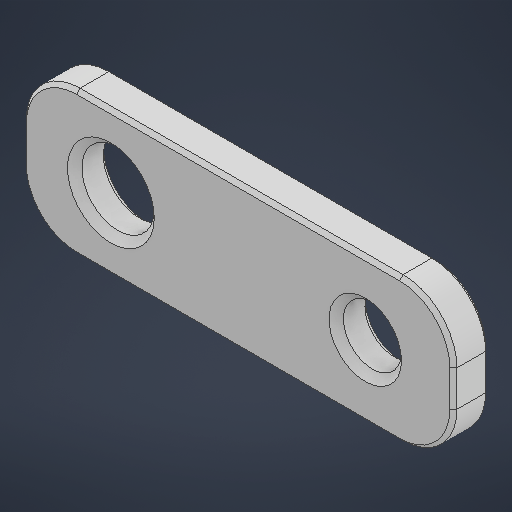
# Autodesk Inventor part: genivaBottom
Saved by Autodesk Inventor 2026.3 (Build 303398000, 398)
## iProperties
Created: 2026-04-30
Part Number: genivaBottom
Material: Generic
Document SubType Name: Modeling
Designer: frede
Density: 1 g/cm^3
Appearance: Default
Author: frede
Autodesk Inventor part; units mm, degrees
ref_plane "YZ Plane" through (0, 0, 0) normal (1, 0, 0) x (0, 1, 0)
ref_plane "XZ Plane" through (0, 0, 0) normal (0, 1, 0) x (-1, 0, 0)
ref_plane "XY Plane" through (0, 0, 0) normal (0, 0, 1) x (1, 0, 0)
sketch "Sketch1" plane through (0, 0, 0) normal (0, 0, 1) x (1, 0, 0)
  circle A0 centre (0, 0) radius 5.05
  circle A1 centre (35.45, 0) radius 4.05
  line L0 (0, 0) -> (35.45, 0)
  line L1 (40.225, 10) -> (-4.775, 10)
  line L2 (-12.275, 2.5) -> (-12.275, -2.5)
  line L3 (-4.775, -10) -> (40.225, -10)
  line L4 (47.725, -2.5) -> (47.725, 2.5)
  line L5 (47.725, 10) -> (-12.275, -10) construction
  line L6 (-12.275, 10) -> (47.725, -10) construction
  arc A2 (-4.775, 10) -> (-12.275, 2.5) centre (-4.775, 2.5) ccw
  arc A3 (47.725, 2.5) -> (40.225, 10) centre (40.225, 2.5) ccw
  arc A4 (40.225, -10) -> (47.725, -2.5) centre (40.225, -2.5) ccw
  arc A5 (-12.275, -2.5) -> (-4.775, -10) centre (-4.775, -2.5) ccw
  point P0 (17.725, 0)
  dimension "d0" = 10.1
  dimension "d1" = 8.1
  dimension "d2" = 60
  dimension "d3" = 20
  dimension "d4" = 7.5
  constraints: 14 end point, 8 point on circle, 8 point on line, 8 tangent, 6 centre point, 3 equal radius, 3 midpoint, 2 horizontal, 2 parallel, 1 coincident, 1 perpendicular
  measures "d0" diameter of A0
  measures "d1" diameter of A1
  measures "d2" distance of L6.end L5.end
  measures "d3" distance of L5.end L6.start
  measures "d4" radius of A2
extrude "Extrusion1" add sketch "Sketch1" along normal blind 5
chamfer "Chamfer1" distance 0.5 angle 45 16 edges at (17.725, 10, 5) (-10.0783, 7.8033, 5) (-12.275, 0, 5) (-10.0783, -7.8033, 5) (17.725, -10, 5) (45.5283, -7.8033, 5) (47.725, 0, 5) (45.5283, 7.8033, 5) (17.725, 10, 0) (-10.0783, 7.8033, 0) (-12.275, 0, 0) (-10.0783, -7.8033, 0) (17.725, -10, 0) (45.5283, -7.8033, 0) (47.725, 0, 0) (45.5283, 7.8033, 0)
chamfer "Chamfer2" distance 1 angle 45 4 edges at (-5.05, 0, 5) (-5.05, 0, 0) (31.4, 0, 5) (31.4, 0, 0)
body "Solid1"
